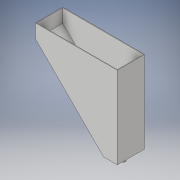
# Autodesk Inventor part: hopper 2
Saved by Autodesk Inventor 2019 (Build 230136000, 136)
## iProperties
Created: 2020-02-12
Part Number: hopper 2
Material: Generic
Document SubType Name: Sheet Metal
Designer: ASUS
Density: 1 g/cm^3
Appearance: Default
Sheet Metal Rule: Default
Author: ASUS
Autodesk Inventor part; units mm, degrees
ref_plane "YZ Plane" through (0, 0, 0) normal (1, 0, 0) x (0, 1, 0)
ref_plane "XZ Plane" through (0, 0, 0) normal (0, 1, 0) x (-1, 0, 0)
ref_plane "XY Plane" through (0, 0, 0) normal (0, 0, 1) x (1, 0, 0)
sketch "Sketch1" plane through (0, 0, 0) normal (0, 1, 0) x (-1, 0, 0)
  line L0 (0, 0) -> (300, 0)
  line L1 (300, 0) -> (300, -100)
  line L2 (300, -100) -> (0, -100)
  line L3 (0, -100) -> (0, 0)
  dimension "d0" = 300
  dimension "d1" = 100
  constraints: 8 end point, 2 parallel, 1 horizontal, 1 perpendicular
  measures "d0" distance of L1.end L2.end
  measures "d1" distance of L0.end L1.end
extrude "Extrusion1" add sketch "Sketch1" along normal blind 300
chamfer "Chamfer1" distance 250 distance2 250 1 edges at (-300, 0, -50) measured on face at (-100, 0, -33.3333)
shell "Shell1" thickness 2 removed faces 1 at (-100, 300, -33.3333)
sketch "Sketch2" plane through (0, 0, 0) normal (0, -1, 0) x (1, 0, 0)
  circle A0 centre (-26.2917, -50) radius 6.35
  point P0 (0, 0)
  dimension "d8" = 12.7
  constraints: 1 centre point
  measures "d8" diameter of A0
extrude "Extrusion2" add sketch "Sketch2" along normal blind 50
sketch "Sketch3" plane through (0, 0, 0) normal (1, 0, 0) x (0, 1, 0)
  circle A0 centre (-44.5235, -49.6457) radius 6.35
  point P0 (0, 0)
  dimension "d11" = 12.7
  constraints: 1 centre point
  measures "d11" diameter of A0
extrude "Extrusion3" add sketch "Sketch3" against normal blind 32 and the other way blind 200
fillet_without_effect "Fillet1"
sketch "Sketch4" plane through (0, 0, 0) normal (0, 0, 1) x (1, 0, 0)
  line L0 (-39.055, -25.4645) -> (218.0396, -25.4645)
  line L1 (218.0396, -25.4645) -> (218.0396, -67.5796)
  line L2 (218.0396, -67.5796) -> (-39.055, -67.5796)
  line L3 (-39.055, -67.5796) -> (-39.055, -25.4645)
  point P0 (0, 0)
  constraints: 8 end point, 2 parallel, 1 horizontal, 1 perpendicular
extrude "Extrusion4" cut sketch "Sketch4" against normal blind 254
equation "\"BendRadius\" = Thickness"
equation "\"BendReliefWidth\" = Thickness"
equation "\"BendReliefDepth\" = 0.5 * Thickness"
equation "\"CornerReliefSize\" = 4 * Thickness"
equation "\"MinimumRemnant\" = 2 * Thickness"
equation "\"TransitionRadius\" = BendRadius"
equation "\"JacobiRadiusSize\" = Thickness"
equation "\"GapSize\" = Thickness"
equation "\"Thickness\" = 3.048"
body "Solid1"
